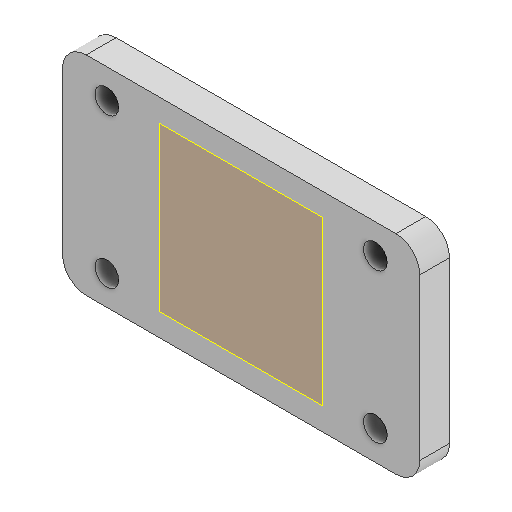
# Autodesk Inventor part: Mold_front_insert_0
Saved by Autodesk Inventor 2022 (Build 260153000, 153)
## iProperties
Created: 2023-03-17
Part Number: Mold_front_insert_0
Material: Generisch
Document SubType Name: Modeling
Designer: diederichbenedict
Density: 1 g/cm^3
Appearance: Vorgabe
Author: diederichbenedict
Autodesk Inventor part; units mm, degrees
ref_plane "YZ Plane" through (0, 0, 0) normal (1, 0, 0) x (0, 1, 0)
ref_plane "XZ Plane" through (0, 0, 0) normal (0, 1, 0) x (-1, 0, 0)
ref_plane "Arbeitsebene1" through (-20.9299, -20.9299, 0) normal (0, 0, 1) x (1, 0, 0)
sketch "Skizze1" plane through (-20.9299, -20.9299, 0) normal (0, 0, 1) x (1, 0, 0)
  line L0 (20.9299, -14.0701) -> (20.9299, 18.6776) construction
  arc A0 (20.9299, 18.6776) -> (20.396, 18.5231) centre (20.9299, 17.6776) ccw construction
  line L1 (20.396, 18.5231) -> (14.9332, 15.0736) construction
  arc A1 (13.0645, 18.033) -> (14.9332, 15.0736) centre (13.9988, 16.5533) ccw construction
  line L2 (13.0645, 18.033) -> (16.3132, 20.0844) construction
  arc A2 (16.3132, 20.0844) -> (16.3132, 21.7755) centre (15.7793, 20.9299) ccw construction
  line L3 (16.3132, 21.7755) -> (13.0645, 23.8269) construction
  arc A3 (14.9332, 26.7863) -> (13.0645, 23.8269) centre (13.9988, 25.3066) ccw construction
  line L4 (14.9332, 26.7863) -> (20.396, 23.3368) construction
  arc A4 (20.396, 23.3368) -> (21.4638, 23.3368) centre (20.9299, 24.1823) ccw construction
  line L5 (21.4638, 23.3368) -> (26.9267, 26.7863) construction
  arc A5 (28.7954, 23.8269) -> (26.9267, 26.7863) centre (27.861, 25.3066) ccw construction
  line L6 (28.7954, 23.8269) -> (25.5466, 21.7755) construction
  arc A6 (25.5466, 21.7755) -> (25.0805, 20.9299) centre (26.0805, 20.9299) ccw construction
  line L7 (25.0805, 20.9299) -> (68.3299, 20.9299) construction
  arc A7 (73.5299, 20.9299) -> (68.3299, 20.9299) centre (70.9299, 20.9299) ccw construction
  line L8 (73.5299, 20.9299) -> (80.9299, 20.9299) construction
  line L9 (80.9299, 20.9299) -> (80.9299, 47.9299) construction
  arc A8 (80.9299, 47.9299) -> (72.9299, 55.9299) centre (72.9299, 47.9299) ccw construction
  line L10 (72.9299, 55.9299) -> (-31.0701, 55.9299) construction
  arc A9 (-31.0701, 55.9299) -> (-39.0701, 47.9299) centre (-31.0701, 47.9299) ccw construction
  line L11 (-39.0701, 47.9299) -> (-39.0701, -6.0701) construction
  arc A10 (-39.0701, -6.0701) -> (-31.0701, -14.0701) centre (-31.0701, -6.0701) ccw construction
  line L12 (-31.0701, -14.0701) -> (20.9299, -14.0701) construction
  circle A11 centre (66.0304, 46.0304) radius 4.5 construction
  line L13 (39.6792, 34.7549) -> (74.3619, 34.7549) construction
  line L14 (74.3619, 34.7549) -> (74.3619, 33.2249) construction
  line L15 (74.3619, 33.2249) -> (39.6792, 33.2249) construction
  arc A12 (37.6256, 34.6486) -> (39.6792, 33.2249) centre (39.6792, 35.4179) ccw construction
  arc A13 (37.6256, 34.6486) -> (32.6949, 33.7349) centre (35.2449, 33.7349) ccw construction
  line L16 (32.6949, 33.7349) -> (32.6949, 28.1249) construction
  arc A14 (32.6949, 28.1249) -> (35.2449, 25.5749) centre (35.2449, 28.1249) ccw construction
  arc A15 (35.2449, 25.5749) -> (37.629, 27.2201) centre (35.2449, 28.1249) ccw construction
  arc A16 (39.6792, 28.6349) -> (37.629, 27.2201) centre (39.6793, 26.4419) ccw construction
  line L17 (39.6792, 28.6349) -> (39.8859, 28.6349) construction
  line L18 (39.8859, 28.6349) -> (74.3619, 28.6349) construction
  line L19 (74.3619, 28.6349) -> (74.3619, 27.1049) construction
  line L20 (74.3619, 27.1049) -> (39.6792, 27.1049) construction
  arc A17 (39.6792, 27.1049) -> (39.0618, 26.6833) centre (39.6792, 26.4419) ccw construction
  arc A18 (31.1649, 28.1249) -> (39.0618, 26.6833) centre (35.2449, 28.1249) ccw construction
  line L21 (31.1649, 28.1249) -> (31.1649, 33.7349) construction
  arc A19 (39.0618, 35.1765) -> (31.1649, 33.7349) centre (35.2449, 33.7349) ccw construction
  arc A20 (39.0618, 35.1765) -> (39.6792, 34.7549) centre (39.6792, 35.4179) ccw construction
  line L22 (2.1806, 27.1049) -> (-32.5021, 27.1049) construction
  line L23 (-32.5021, 27.1049) -> (-32.5021, 28.6349) construction
  line L24 (-32.5021, 28.6349) -> (2.1806, 28.6349) construction
  arc A21 (4.2342, 27.2113) -> (2.1806, 28.6349) centre (2.1806, 26.4419) ccw construction
  arc A22 (4.2342, 27.2113) -> (9.1649, 28.1249) centre (6.6149, 28.1249) ccw construction
  line L25 (9.1649, 28.1249) -> (9.1649, 33.7349) construction
  arc A23 (9.1649, 33.7349) -> (6.6149, 36.2849) centre (6.6149, 33.7349) ccw construction
  arc A24 (6.6149, 36.2849) -> (4.2309, 34.6398) centre (6.6149, 33.7349) ccw construction
  arc A25 (2.1806, 33.2249) -> (4.2309, 34.6398) centre (2.1806, 35.4179) ccw construction
  line L26 (2.1806, 33.2249) -> (1.9739, 33.2249) construction
  line L27 (1.9739, 33.2249) -> (-32.5021, 33.2249) construction
  line L28 (-32.5021, 33.2249) -> (-32.5021, 34.7549) construction
  line L29 (-32.5021, 34.7549) -> (2.1806, 34.7549) construction
  arc A26 (2.1806, 34.7549) -> (2.7981, 35.1765) centre (2.1806, 35.4179) ccw construction
  arc A27 (10.6949, 33.7349) -> (2.7981, 35.1765) centre (6.6149, 33.7349) ccw construction
  line L30 (10.6949, 33.7349) -> (10.6949, 28.1249) construction
  arc A28 (2.7981, 26.6833) -> (10.6949, 28.1249) centre (6.6149, 28.1249) ccw construction
  arc A29 (2.7981, 26.6833) -> (2.1806, 27.1049) centre (2.1806, 26.4419) ccw construction
  line L31 (2.1806, 7.1049) -> (-32.5021, 7.1049) construction
  line L32 (-32.5021, 7.1049) -> (-32.5021, 8.6349) construction
  line L33 (-32.5021, 8.6349) -> (2.1806, 8.6349) construction
  arc A30 (4.2342, 7.2113) -> (2.1806, 8.6349) centre (2.1806, 6.4419) ccw construction
  arc A31 (4.2342, 7.2113) -> (9.1649, 8.1249) centre (6.6149, 8.1249) ccw construction
  line L34 (9.1649, 8.1249) -> (9.1649, 13.7349) construction
  arc A32 (9.1649, 13.7349) -> (6.6149, 16.2849) centre (6.6149, 13.7349) ccw construction
  arc A33 (6.6149, 16.2849) -> (4.2309, 14.6398) centre (6.6149, 13.7349) ccw construction
  arc A34 (2.1806, 13.2249) -> (4.2309, 14.6398) centre (2.1806, 15.4179) ccw construction
  line L35 (2.1806, 13.2249) -> (1.9739, 13.2249) construction
  line L36 (1.9739, 13.2249) -> (-32.5021, 13.2249) construction
  line L37 (-32.5021, 13.2249) -> (-32.5021, 14.7549) construction
  line L38 (-32.5021, 14.7549) -> (2.1806, 14.7549) construction
  arc A35 (2.1806, 14.7549) -> (2.7981, 15.1765) centre (2.1806, 15.4179) ccw construction
  arc A36 (10.6949, 13.7349) -> (2.7981, 15.1765) centre (6.6149, 13.7349) ccw construction
  line L39 (10.6949, 13.7349) -> (10.6949, 8.1249) construction
  arc A37 (2.7981, 6.6833) -> (10.6949, 8.1249) centre (6.6149, 8.1249) ccw construction
  arc A38 (2.7981, 6.6833) -> (2.1806, 7.1049) centre (2.1806, 6.4419) ccw construction
  circle A39 centre (-24.1706, -4.1706) radius 4.5 construction
  circle A40 centre (-24.1706, 46.0304) radius 4.5 construction
  circle A41 centre (-29.0701, 20.9299) radius 2.6 construction
  circle A42 centre (-24.1706, 46.0304) radius 4 construction
  circle A43 centre (66.0304, 46.0304) radius 4 construction
  circle A44 centre (-24.1706, -4.1706) radius 4 construction
  line L40 (-31.0701, 55.9299) -> (72.9299, 55.9299)
  line L41 (80.9299, 47.9299) -> (80.9299, -6.0701)
  line L42 (72.9299, -14.0701) -> (-31.0701, -14.0701)
  line L43 (-39.0701, -6.0701) -> (-39.0701, 47.9299)
  circle A45 centre (-24.1706, 46.0304) radius 4
  circle A46 centre (66.0304, 46.0304) radius 4
  circle A47 centre (-24.1706, -4.1706) radius 4
  circle A48 centre (66.0304, -4.1706) radius 4
  arc A49 (-31.0701, 55.9299) -> (-39.0701, 47.9299) centre (-31.0701, 47.9299) ccw
  arc A50 (80.9299, 47.9299) -> (72.9299, 55.9299) centre (72.9299, 47.9299) ccw
  arc A51 (72.9299, -14.0701) -> (80.9299, -6.0701) centre (72.9299, -6.0701) ccw
  arc A52 (-39.0701, -6.0701) -> (-31.0701, -14.0701) centre (-31.0701, -6.0701) ccw
  point P0 (20.9299, 20.9299)
  dimension "d0" = 8
  constraints: 8 centre point, 8 end point, 8 point on circle, 8 tangent, 6 equal radius, 3 coincident, 2 parallel, 1 horizontal, 1 perpendicular
  measures "d0" radius of A49
ref_plane "Arbeitsebene2" through (-60, -35, -10) normal (0, 0, -1) x (0, 1, 0)
extrude "Extrusion1" add sketch "Skizze1" against normal up to surface (10 mm away)
